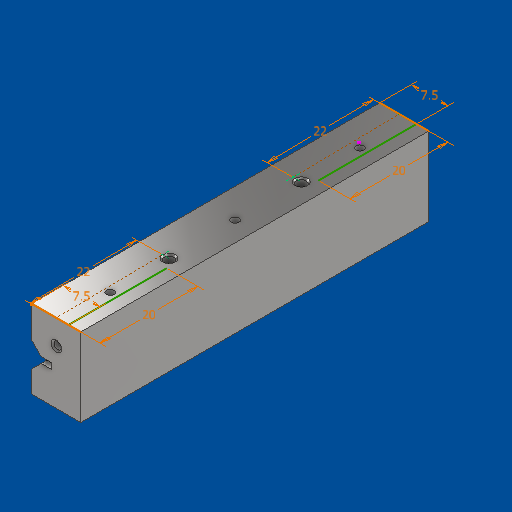
# Autodesk Inventor part: Guide
Saved by Autodesk Inventor 2025.1 (Build 291241000, 241)
## iProperties
Created: 2024-12-11
Part Number: Guide
Material: Steel, Carbon
Document SubType Name: Modeling
Designer: konch
Density: 7.85 g/cm^3
Appearance: Semi-Polished
Mass: 11.3965 g
Surface Area: 49.0354 cm^2
Volume: 11.3965 cm^3
Description: C55
Author: konch
Autodesk Inventor part; units mm, degrees
ref_plane "YZ Plane" through (0, 0, 0) normal (1, 0, 0) x (0, 1, 0)
ref_plane "XZ Plane" through (0, 0, 0) normal (0, 1, 0) x (-1, 0, 0)
ref_plane "XY Plane" through (0, 0, 0) normal (0, 0, 1) x (1, 0, 0)
sketch "Sketch1" plane through (0, 0, 0) normal (0, 0, 1) x (1, 0, 0)
  line L0 (0, 0) -> (0, 5.657)
  line L1 (2.8285, 3.4285) -> (2.2285, 3.4285)
  line L2 (2.8285, 2.2285) -> (2.2285, 2.2285)
  line L3 (2.2285, 3.4285) -> (2.8285, 3.4285)
  line L4 (2.8285, 2.2285) -> (2.2285, 2.2285)
  line L5 (2.2285, 3.4285) -> (4, 3.4285)
  line L6 (4, 2.2285) -> (2.8285, 2.2285)
  line L7 (2.2285, 3.4285) -> (4, 3.4285)
  line L8 (2.2285, 3.4285) -> (4, 3.4285)
  line L9 (0, -2.1715) -> (0, 0)
  line L10 (0, 5.657) -> (0, 6.8285)
  line L11 (8, -2.1715) -> (8, 6.8285)
  line L12 (4, 3.4285) -> (4, 3.4285)
  line L13 (4, 3.4285) -> (4, 2.2285)
  line L14 (4, 2.2285) -> (4, 2.2285)
  line L15 (8, -2.1715) -> (8, -4.1715)
  line L16 (8, -4.1715) -> (0, -4.1715)
  line L17 (2.2285, 3.4285) -> (1.9283, 3.4285)
  line L18 (1.9283, 3.4285) -> (0, 5.3568)
  line L19 (2.2285, 2.2285) -> (1.9283, 2.2285)
  line L20 (1.9283, 2.2285) -> (0, 0.3002)
  line L21 (0, -2.1715) -> (0, -4.1715)
  line L22 (4, 2.8285) -> (8, 2.8285) construction
  line L23 (8, 6.8285) -> (8, 11.8285)
  line L24 (8, 11.8285) -> (0, 11.8285)
  line L25 (0, 11.8285) -> (0, 6.8285)
  line L26 (8, 11.8285) -> (10, 11.8285)
  line L27 (10, 11.8285) -> (10, -4.1715)
  line L28 (10, -4.1715) -> (8, -4.1715)
  line L29 (10, 11.8285) -> (7, 11.8285) construction
  line L30 (10, 11.8285) -> (5, 11.8285) construction
  line L31 (5, 11.8285) -> (5, 6.7848) construction
  point P0 (4.938, 0.6604)
  point P1 (0.4, 0.4)
  point P2 (0.4, 5.257)
  point P3 (0.4, -2.1715)
  point P4 (0.25, 5.407)
  point P5 (0.25, -2.1715)
  point P6 (0.25, -4.1715)
  dimension "d11" = 8
  dimension "d23" = 4
  dimension "d24" = 7
  dimension "d25" = 5
  dimension "d26" = 2
  dimension "d29" = 5
  dimension "d78" = 4
  constraints: 64 end point, 10 perpendicular, 6 point on line, 4 vertical, 3 horizontal, 1 coincident, 1 collinear, 1 midpoint
  measures "d11" distance of L11.end L10.end
  measures "d23" distance of L11.end L22.end
  measures "d24" distance of L22.end L15.end
  measures "d25" distance of L11.end L23.end
  measures "d26" distance of L23.end L26.end
  measures "d29" distance of L26.end L30.end
  measures "d78" distance from line of L9 L22.start
extrude "Extrusion1" add sketch "Sketch1" against normal blind 71 contours L0 L20 L19 L2 L6 L13 L5 L1 L17 L18 L10 L25 L24 L23 L11 L15 L16 L21 L9 | L15 L11 L23 L26 L27 L28
sketch "Sketch2" plane through (0, 0, 0) normal (0, 0, 1) x (1, 0, 0)
  line L0 (10, -4.1715) -> (10, 11.8285) construction
  line L1 (10, 11.8285) -> (5, 11.8285) construction
  line L2 (10, 11.8285) -> (0, 11.8285) construction
  line L3 (5, 11.8285) -> (5, 6.8285) construction
  point P0 (0, 0)
  dimension "d30" = 5
  constraints: 4 end point, 1 coincident, 1 midpoint, 1 perpendicular
  measures "d30" distance of L1.end L3.end
hole "Hole1" at (5, 6.8285, 0) direction (0, 0, -1) diameter 1.567 depth 8 tip angle 118 thread size "M2x0.4" class "6H" standard "ANSI Metric M Profile"
sketch "Sketch3" plane through (0, 0, -71) normal (0, 0, -1) x (-1, 0, 0)
  line L0 (-10, 11.8285) -> (-10, -4.1715) construction
  line L1 (-10, 11.8285) -> (-5, 11.8285) construction
  line L2 (0, 11.8285) -> (-10, 11.8285) construction
  line L3 (-5, 11.8285) -> (-5, 6.8285) construction
  circle A0 centre (-5, 6.8285) radius 0.7835 construction
  point P0 (0, 0)
  dimension "d38" = 5
  dimension "d40" = 5
  constraints: 4 end point, 1 coincident, 1 midpoint, 1 perpendicular
  measures "d38" distance of L0.start L1.end
  measures "d40" distance of L1.end L3.end
hole "Hole2" at (5, 6.8285, -71) direction (0, 0, 1) diameter 1.567 depth 8 tip angle 118 thread size "M2x0.4" class "6H" standard "ISO Metric profile"
chamfer "Chamfer1" distance 0.3 angle 45 1 edges at (5, 7.612, 0)
chamfer "Chamfer2" distance 0.3 angle 45 1 edges at (5, 6.045, -71)
sketch "Sketch4" plane through (0, -4.1715, 0) normal (0, -1, 0) x (1, 0, 0)
  line L0 (0, 0) -> (0, -71) construction
  line L1 (0, 0) -> (0, -10) construction
  line L2 (0, -10) -> (0, -35.5) construction
  line L3 (0, -71) -> (0, -61) construction
  line L4 (0, -35.5) -> (10, -35.5) construction
  line L5 (10, 0) -> (10, -71) construction
  line L6 (0, -61) -> (10, -61) construction
  line L7 (0, -10) -> (10, -10) construction
  line L8 (0, -71) -> (6, -71)
  line L9 (6, -71) -> (6, 0)
  point P0 (5, 0)
  point P1 (5, -71)
  point P2 (6, -61)
  point P3 (6, -35.5)
  point P4 (6, -10)
  dimension "d54" = 10
  dimension "d55" = 10
  dimension "d63" = 6
  dimension "d64" = 35.5
  constraints: 16 end point, 8 point on line, 4 perpendicular, 3 midpoint
  measures "d54" distance of L0.start L1.end
  measures "d55" distance of L0.end L3.end
  measures "d63" distance of L0.end L8.end
  measures "d64" distance from line of L8 point (6, -35.5)
hole "Hole3" at (6, -4.1715, -10) at (6, -4.1715, -35.5) at (6, -4.1715, -61) direction (0, 1, 0) diameter 1.567 end through all thread size "M2x0.4" class "6H" standard "ISO Metric profile"
sketch "Sketch5" plane through (0, 11.8285, 0) normal (0, 1, 0) x (1, 0, 0)
  point P0 (0, 0)
chamfer "Chamfer3" distance 0.3 angle 45 1 edges at (6, -4.1715, -9.2165)
chamfer "Chamfer4" distance 0.3 angle 45 2 edges at (6, -4.1715, -34.7165) (6, -4.1715, -60.2165)
sketch "Sketch6" plane through (0, 11.8285, 0) normal (0, 1, 0) x (1, 0, 0)
  line L0 (0, 0) -> (10, 0) projected
  line L1 (4, 71) -> (4.3098, 49.0022) construction
  line L2 (5, 0) -> (4.6902, 21.9978) construction
  point P0 (5, 61.7835)
  dimension "d71" = 22
  dimension "d72" = 22
  constraints: 4 end point, 2 coincident, 1 midpoint
  measures "d71" distance of L1.start L1.end
  measures "d72" distance of L2.start L2.end
sketch "Sketch7" plane through (0, 11.8285, 0) normal (0, 1, 0) x (1, 0, 0)
  line L0 (0, 0) -> (10, 0) projected
  line L1 (0, 0) -> (7.5, 0)
  line L2 (7.5, 0) -> (7.5, 20)
  line L3 (0, 71) -> (10, 71) projected
  line L4 (0, 71) -> (7.5, 71)
  line L5 (7.5, 71) -> (7.5, 51)
  dimension "d73" = 7.5
  dimension "d74" = 20
  dimension "d76" = 7.5
  dimension "d77" = 20
  constraints: 8 end point, 2 perpendicular, 2 point on line
  measures "d73" distance of L0.start L1.end
  measures "d74" distance of L1.end L2.end
  measures "d76" distance of L3.start L4.end
  measures "d77" distance of L4.end L5.end
sketch "Sketch8" plane through (0, 11.8285, 0) normal (0, 1, 0) x (1, 0, 0)
  line L0 (0, 0) -> (6, 0)
  line L1 (10, 0) -> (0, 0) projected
  line L2 (6, 0) -> (6, 22)
  line L3 (0, 71) -> (6, 71)
  line L4 (10, 71) -> (0, 71) projected
  line L5 (6, 71) -> (6, 49)
  dimension "d79" = 6
  dimension "d80" = 22
  dimension "d81" = 6
  dimension "d82" = 22
  constraints: 8 end point, 2 coincident, 2 perpendicular, 2 point on line
  measures "d79" distance of L0.start L0.end
  measures "d80" distance of L0.end L2.end
  measures "d81" distance of L3.start L3.end
  measures "d82" distance of L3.end L5.end
hole "Hole4" at (6, 11.8285, -49) at (6, 11.8285, -22) direction (0, -1, 0) diameter 2 end through all
chamfer "Chamfer5" distance 0.3 angle 45 2 edges at (6, 11.8285, -50) (6, 11.8285, -23)
body "Solid1"
